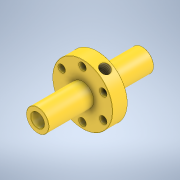
# Autodesk Inventor part: Anode
Saved by Autodesk Inventor 2020 (Build 240168000, 168)
## iProperties
Created: 2019-09-29
Part Number: Anode
Material: Copper
Document SubType Name: Modeling
Designer: vmiguel
Density: 8.94 g/cm^3
Appearance: Glossy - Gold
Author: vmiguel
Autodesk Inventor part; units mm, degrees
ref_plane "XZ Plane" through (0, 0, 0) normal (0, 1, 0) x (-1, 0, 0)
ref_plane "XY Plane" through (0, 0, 0) normal (0, 0, 1) x (1, 0, 0)
sketch "Sketch1" plane through (0, 0, 0) normal (1, 0, 0) x (0, 1, 0)
  line L0 (0, 0) -> (0, -33.1818)
  line L1 (4.5, 10.1062) -> (20, 10.1062)
  line L2 (20, 10.1062) -> (20, 0.1062)
  line L3 (20, 0.1062) -> (7.5, 0.1062)
  line L4 (7.5, 0.1062) -> (7.5, -29.8938)
  line L5 (7.5, -29.8938) -> (4.5, -29.8938)
  line L6 (4.5, -29.8938) -> (4.5, 10.1062)
  line L7 (7.5, 10.1062) -> (7.5, 40.1062)
  line L8 (7.5, 40.1062) -> (4.5, 40.1062)
  line L9 (4.5, 40.1062) -> (4.5, 10.1062)
  dimension "d0" = 9
  dimension "d1" = 15
  dimension "d2" = 30
  dimension "d3" = 10
  dimension "d4" = 40
  dimension "d28" = 30
  constraints: 21 end point, 7 perpendicular, 2 vertical, 1 horizontal, 1 point on line
  measures "d0" diameter of L6 L0
  measures "d1" diameter of L4 L0
  measures "d2" distance of L3.end L4.end
  measures "d3" distance of L1.end L2.end
  measures "d4" diameter of L2 L0
  measures "d28" distance of L7.start L7.end
revolve "Revolution1" add sketch "Sketch1" angle 360 about axis through (0, 0, 0) along (0, 0, -1)
sketch "Sketch2" plane through (0, 0, 10.1062) normal (0, 0, 1) x (1, 0, 0)
  point P0 (0, 0)
  point P1 (0, 16)
  dimension "d6" = 16
  constraints: 1 vertical alignment
  measures "d6" distance of point (0, 16) point (0, 0)
hole "Hole1" at (0, 16, 10.1062) direction (0, 0, -1) diameter 5 end through all
pattern_circular "Circular Pattern1" count 6 over 360 about axis through (0, 0, 5.1062) along (0, 0, -1) of "Hole1"
ref_plane "Work Plane2" through (10, 17.3205, 5.1062) normal (0.5, 0.866, 0) x (-0.866, 0.5, 0)
ref_plane "Work Plane1" through (0, 0, 0) normal (0.5, 0.866, 0) x (0, 0, 1)
sketch "Sketch3" plane through (10, 17.3205, 5.1062) normal (0.5, 0.866, 0) x (-0.866, 0.5, 0)
  line L0 (-20, 5) -> (20, 5) projected
  line L1 (-20, -5) -> (20, -5) projected
  line L2 (0, 5) -> (0, -5.1062)
  point P0 (0, -0.0531)
  constraints: 2 end point, 2 midpoint, 1 vertical
hole "Hole2" at (10, 17.3205, 5.0531) direction (-0.5, -0.866, 0) diameter 6.647 depth 20.2 tip angle 118 thread size "M8x1.25" class "6H" standard "ANSI Metric M Profile"
chamfer "Chamfer1" distance 0.2 angle 45 5 edges at (0, -20, 0.1062) (0, -20, 10.1062) (0, -7.5, -29.8938) (0, -7.5, 40.1062) (0, -4.5, 40.1062)
equation "\"d28\" = d2"
body "Solid1"
